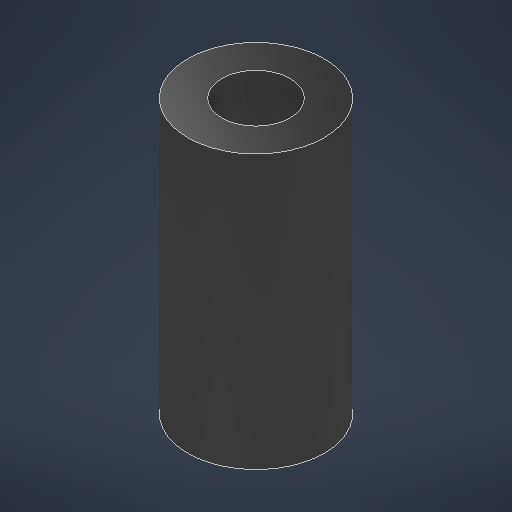
# Autodesk Inventor part: Abstandsbolzen PA6.0 schwarz Ø6x12 Gewinde M3 durchgehend
Saved by Autodesk Inventor 2026.1 (Build 301233020, 233B)
## iProperties
Created: 2026-04-17
Part Number: Abstandsbolzen PA6.0 schwarz Ø6x12 Gewinde M3 durchgehend
Material: Generic
Document SubType Name: Modeling
Designer: Bahaa
Mass: 0.254469 g
Surface Area: 3.81704 cm^2
Volume: 0.254469 cm^3
Density: 1 g/cm^3
Appearance: Glossy - Black
Author: Bahaa
Autodesk Inventor part; units mm, degrees
ref_plane "YZ Plane" through (0, 0, 0) normal (1, 0, 0) x (0, 1, 0)
ref_plane "XZ Plane" through (0, 0, 0) normal (0, 1, 0) x (-1, 0, 0)
ref_plane "XY Plane" through (0, 0, 0) normal (0, 0, 1) x (1, 0, 0)
sketch "Sketch1" plane through (0, 0, 0) normal (0, 0, 1) x (1, 0, 0)
  circle A0 centre (0, 0) radius 3
  circle A1 centre (0, 0) radius 1.5
  dimension "d0" = 6
  dimension "d1" = 3
  constraints: 2 centre point, 2 coincident
  measures "d0" diameter of A0
  measures "d1" diameter of A1
extrude "Extrusion1" add sketch "Sketch1" along normal blind 12
body "Solid1"
